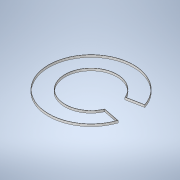
# Autodesk Inventor part: Level 2 Edge Banding
Saved by Autodesk Inventor 2020 (Build 240168000, 168)
## iProperties
Created: 2020-07-30
Part Number: Level 2 Edge Banding
Material: Generic
Document SubType Name: Modeling
Designer: Dan Wikman
Density: 1 g/cm^3
Appearance: Default
Author: Dan Wikman
Autodesk Inventor part; units mm, degrees
ref_plane "YZ Plane" through (0, 0, 0) normal (1, 0, 0) x (0, 1, 0)
ref_plane "XZ Plane" through (0, 0, 0) normal (0, 1, 0) x (-1, 0, 0)
ref_plane "XY Plane" through (0, 0, 0) normal (0, 0, 1) x (1, 0, 0)
sketch "Sketch1" plane through (0, 0, 0) normal (0, 1, 0) x (-1, 0, 0)
  line L0 (-545.8153, 185.3726) -> (-326.5965, 142.7608)
  line L1 (-545.8153, -185.3726) -> (-326.5965, -142.7608)
  arc A0 (-545.8153, -185.3726) -> (-545.8153, 185.3726) centre (0, 0) ccw
  arc A1 (-326.5965, -142.7608) -> (-326.5965, 142.7608) centre (0, 0) ccw
  arc A2 (-324.2, -138.2201) -> (-324.2, 138.2201) centre (0, 0) ccw
  arc A3 (-551.0584, -182.3169) -> (-551.0584, 182.3169) centre (0, 0) ccw
  line L2 (-551.0584, 182.3169) -> (-324.2, 138.2201)
  line L3 (-324.2, -138.2201) -> (-551.0584, -182.3169)
  dimension "d81" = 4
  dimension "d82" = 4
  constraints: 8 end point, 8 point on circle, 4 centre point, 3 coincident, 1 parallel
  measures "d81" distance between parallel lines of L0 L2
  measures "d82" distance between parallel lines of L1 L3
extrude "Extrusion2" add sketch "Sketch1" along normal blind 30
body "Solid2"
